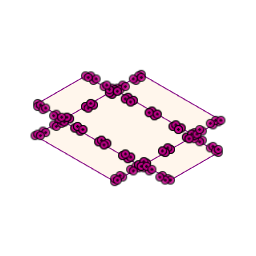
3dBox v7 (Autodesk Fusion 360 design; units mm, degrees)
Autodesk Fusion 360 part; units mm, degrees
sketch "Sketch1" plane through (0, 0, 0) normal (0, 0, 1) x (1, 0, 0) in component "bottom"
  line L0 (0, 100) -> (150, 100)
  line L1 (150, 100) -> (150, 0)
  line L2 (150, 0) -> (0, 0)
  line L3 (0, 0) -> (0, 100)
  line L4 (150, 100) -> (145, 100)
  line L5 (145, 100) -> (145, 90)
  line L6 (145, 90) -> (150, 90)
  line L7 (150, 90) -> (150, 55)
  line L8 (150, 55) -> (145, 55)
  line L9 (145, 55) -> (145, 45)
  line L10 (145, 45) -> (150, 45)
  line L11 (150, 45) -> (150, 10)
  line L12 (150, 10) -> (145, 10)
  line L13 (145, 10) -> (145, 0)
  line L14 (145, 0) -> (150, 0)
  line L15 (75, 100) -> (75, 0) construction
  line L16 (5, 100) -> (5, 90)
  line L17 (5, 90) -> (0, 90)
  line L18 (0, 55) -> (5, 55)
  line L19 (5, 55) -> (5, 45)
  line L20 (5, 45) -> (0, 45)
  line L21 (0, 10) -> (5, 10)
  line L22 (5, 10) -> (5, 0)
  line L23 (5, 0) -> (0, 0)
  line L24 (25, 100) -> (25, 95)
  line L25 (25, 95) -> (35, 95)
  line L26 (35, 95) -> (35, 100)
  line L27 (35, 100) -> (70, 100)
  line L28 (70, 100) -> (70, 95)
  line L29 (70, 95) -> (80, 95)
  line L30 (80, 95) -> (80, 100)
  line L31 (80, 100) -> (115, 100)
  line L32 (115, 100) -> (115, 95)
  line L33 (115, 95) -> (125, 95)
  line L34 (125, 95) -> (125, 100)
  line L35 (125, 100) -> (145, 100)
  line L36 (25, 100) -> (5, 100)
  line L37 (75, 50) -> (103.6625, 50) construction
  line L38 (25, 0) -> (25, 5)
  line L39 (25, 5) -> (35, 5)
  line L40 (35, 5) -> (35, 0)
  line L41 (70, 0) -> (70, 5)
  line L42 (70, 5) -> (80, 5)
  line L43 (80, 5) -> (80, 0)
  line L44 (115, 0) -> (115, 5)
  line L45 (115, 5) -> (125, 5)
  line L46 (125, 5) -> (125, 0)
  dimension "d1" = 150
  dimension "d2" = 100
  dimension "d5" = 5
  dimension "d6" = 5
  dimension "d7" = 5
  dimension "d8" = 5
  dimension "d9" = 5
  dimension "d10" = 5
  dimension "d11" = 100
  dimension "d12" = 10
  dimension "d13" = 10
  dimension "d14" = 10
  dimension "d15" = 5
  dimension "d16" = 5
  dimension "d17" = 5
  dimension "d18" = 5
  dimension "d19" = 5
  dimension "d20" = 5
  dimension "d21" = 10
  dimension "d22" = 10
  dimension "d23" = 10
  dimension "d24" = 140
  dimension "d25" = 20
  dimension "d26" = 20
  constraint horizontal L0
  constraint vertical L1
  constraint horizontal L2
  constraint vertical L3
  constraint coincident L2.end L3.start
  constraint horizontal L4
  constraint perpendicular L4 L5
  constraint perpendicular L5 L6
  constraint perpendicular L6 L7
  constraint perpendicular L7 L8
  constraint perpendicular L8 L9
  constraint perpendicular L7 L10
  constraint perpendicular L8 L11
  constraint perpendicular L11 L12
  constraint perpendicular L12 L13
  constraint perpendicular L13 L14
  constraint equal L7 L11
  constraint coincident L1.end L2.start
  constraint midpoint L0 L15.start
  constraint midpoint L2 L15.end
  constraint symmetric L4.end L15 L16.start
  constraint symmetric L5.end L15 L16.end
  constraint symmetric L6.end L15 L17.end
  constraint symmetric L7.end L15 L18.start
  constraint symmetric L8.end L15 L18.end
  constraint symmetric L9.end L15 L19.end
  constraint symmetric L10.end L15 L20.end
  constraint symmetric L11.end L15 L21.start
  constraint symmetric L12.end L15 L21.end
  constraint symmetric L13.end L15 L22.end
  constraint symmetric L1.end L15 L2.end
  constraint perpendicular L0 L24
  constraint perpendicular L24 L25
  constraint perpendicular L25 L26
  constraint perpendicular L26 L27
  constraint perpendicular L27 L28
  constraint perpendicular L28 L29
  constraint perpendicular L29 L30
  constraint perpendicular L30 L31
  constraint perpendicular L31 L32
  constraint perpendicular L30 L33
  constraint perpendicular L33 L34
  constraint perpendicular L34 L35
  constraint perpendicular L24 L36
  constraint equal L27 L31
  constraint coincident L16.start L36.end
  constraint midpoint L15 L37.start
  constraint perpendicular L1 L37
  constraint symmetric L24.start L37 L38.start
  constraint symmetric L24.end L37 L38.end
  constraint symmetric L25.end L37 L39.end
  constraint symmetric L26.end L37 L40.end
  constraint symmetric L27.end L37 L41.start
  constraint symmetric L28.end L37 L41.end
  constraint symmetric L29.end L37 L42.end
  constraint symmetric L30.end L37 L43.end
  constraint symmetric L31.end L37 L44.start
  constraint symmetric L32.end L37 L44.end
  constraint symmetric L33.end L37 L45.end
  constraint symmetric L34.end L37 L46.end
  measures "d1" distance of L0.start L0.end
  measures "d2" distance of L0.start L2.end
  measures "d5" distance of L0.end L4.end
  measures "d6" distance of L5.end L6.end
  measures "d7" distance of L7.end L8.end
  measures "d8" distance of L9.end L10.end
  measures "d9" distance of L11.end L12.end
  measures "d10" distance of L13.end L1.end
  measures "d11" distance of L0.end L1.end
  measures "d12" distance of L12.end L13.end
  measures "d13" distance of L8.end L9.end
  measures "d14" distance of L4.end L5.end
  measures "d15" distance of L33.end L34.end
  measures "d16" distance of L31.end L32.end
  measures "d17" distance of L29.end L30.end
  measures "d18" distance of L27.end L28.end
  measures "d19" distance of L25.end L26.end
  measures "d20" distance of L24.start L24.end
  measures "d21" distance of L24.end L25.end
  measures "d22" distance of L28.end L29.end
  measures "d23" distance of L32.end L33.end
  measures "d24" distance of L4.end L16.start
  measures "d25" distance of L34.end L4.end
  measures "d26" distance of L24.start L16.start
extrude "Extrude1" add sketch "Sketch1" along normal blind 5 contours L0 L1 L2 L3 L5 L6 L7 L8 L9 L10 L11 L12 L13 L16 L17 L18 L19 L20 L21 L22 L24 L25 L26 L27 L28 L29 L30 L31 L32 L33 L34 L35 L36 L38 L39 L40 L41 L42 L43 L44 L45 L46 makes body 1 in component "bottom"
sketch "Sketch1 (2)" plane through (0, 0, 0) normal (0, 0, 1) x (1, 0, 0) in component "sSide"
  line L0 (115, 0) -> (115, 5)
  line L1 (115, 5) -> (125, 5)
  line L2 (125, 5) -> (125, 0)
  line L3 (125, 0) -> (145, 0)
  line L4 (145, 0) -> (145, 10)
  line L5 (145, 10) -> (150, 10)
  line L6 (150, 10) -> (150, 45)
  line L7 (150, 45) -> (145, 45)
  line L8 (145, 45) -> (145, 55)
  line L9 (145, 55) -> (150, 55)
  line L10 (150, 55) -> (150, 90)
  line L11 (150, 90) -> (145, 90)
  line L12 (145, 90) -> (145, 100)
  line L13 (145, 100) -> (125, 100)
  line L14 (125, 100) -> (125, 95)
  line L15 (125, 95) -> (115, 95)
  line L16 (115, 95) -> (115, 100)
  line L17 (115, 100) -> (80, 100)
  line L18 (80, 100) -> (80, 95)
  line L19 (80, 95) -> (70, 95)
  line L20 (70, 95) -> (70, 100)
  line L21 (70, 100) -> (35, 100)
  line L22 (35, 100) -> (35, 95)
  line L23 (35, 95) -> (25, 95)
  line L24 (25, 95) -> (25, 100)
  line L25 (25, 100) -> (5, 100)
  line L26 (5, 100) -> (5, 90)
  line L27 (5, 90) -> (0, 90)
  line L28 (0, 90) -> (0, 55)
  line L29 (0, 55) -> (5, 55)
  line L30 (5, 55) -> (5, 45)
  line L31 (5, 45) -> (0, 45)
  line L32 (0, 45) -> (0, 10)
  line L33 (0, 10) -> (5, 10)
  line L34 (5, 10) -> (5, 0)
  line L35 (5, 0) -> (25, 0)
  line L36 (25, 0) -> (25, 5)
  line L37 (25, 5) -> (35, 5)
  line L38 (35, 5) -> (35, 0)
  line L39 (35, 0) -> (70, 0)
  line L40 (70, 0) -> (70, 5)
  line L41 (70, 5) -> (80, 5)
  line L42 (80, 5) -> (80, 0)
  line L43 (80, 0) -> (115, 0)
  line L44 (145, 100) -> (200, 100)
  line L45 (200, 100) -> (200, 0)
  line L46 (200, 0) -> (145, 0)
  line L47 (145, 100) -> (150, 100)
  line L48 (150, 100) -> (150, 95)
  line L49 (150, 95) -> (155, 95)
  line L50 (155, 95) -> (155, 100)
  line L51 (155, 100) -> (165, 100)
  line L52 (165, 100) -> (165, 95)
  line L53 (165, 95) -> (185, 95)
  line L54 (185, 95) -> (185, 100)
  line L55 (185, 100) -> (195, 100)
  line L56 (195, 100) -> (195, 95)
  line L57 (195, 95) -> (200, 95)
  line L58 (200, 50) -> (169.7246, 50) construction
  line L59 (195, 5) -> (200, 5)
  line L60 (195, 0) -> (195, 5)
  line L61 (185, 5) -> (185, 0)
  line L62 (165, 5) -> (185, 5)
  line L63 (165, 0) -> (165, 5)
  line L64 (155, 5) -> (155, 0)
  line L65 (150, 5) -> (155, 5)
  line L66 (150, 0) -> (150, 5)
  dimension "d55" = 5
  dimension "d56" = 5
  dimension "d57" = 5
  dimension "d58" = 5
  dimension "d59" = 5
  dimension "d60" = 5
  dimension "d61" = 5
  dimension "d62" = 5
  dimension "d63" = 10
  dimension "d64" = 10
  dimension "d65" = 55
  dimension "d66" = 55
  constraint coincident L12.end L13.start
  constraint perpendicular L12 L44
  constraint perpendicular L3 L45
  constraint coincident L3.end L4.start
  constraint perpendicular L4 L46
  constraint horizontal L47
  constraint perpendicular L47 L48
  constraint perpendicular L48 L49
  constraint perpendicular L47 L50
  constraint perpendicular L50 L51
  constraint perpendicular L47 L52
  constraint perpendicular L52 L53
  constraint perpendicular L53 L54
  constraint perpendicular L54 L55
  constraint perpendicular L55 L56
  constraint perpendicular L56 L57
  constraint midpoint L45 L58.start
  constraint perpendicular L45 L58
  constraint symmetric L47.end L58 L66.start
  constraint symmetric L48.end L58 L65.start
  constraint symmetric L49.end L58 L64.start
  constraint symmetric L50.end L58 L64.end
  constraint symmetric L51.end L58 L63.start
  constraint symmetric L52.end L58 L62.start
  constraint symmetric L53.end L58 L61.start
  constraint symmetric L54.end L58 L61.end
  constraint symmetric L55.end L58 L60.start
  constraint symmetric L56.end L58 L59.start
  constraint symmetric L57.end L58 L59.end
  measures "d55" distance of L12.end L47.end
  measures "d56" distance of L47.end L48.end
  measures "d57" distance of L48.end L49.end
  measures "d58" distance of L49.end L50.end
  measures "d59" distance of L51.end L52.end
  measures "d60" distance of L53.end L54.end
  measures "d61" distance of L55.end L56.end
  measures "d62" distance of L56.end L57.end
  measures "d63" distance of L50.end L51.end
  measures "d64" distance of L54.end L55.end
  measures "d65" distance of L12.end L44.end
  measures "d66" horizontal distance of L12.end L57.end
extrude "Extrude1'" add sketch "Sketch1 (2)" along normal blind 5 separate body contours L4 L5 L6 L7 L8 L9 L10 L11 L12 L44 L45 L46 L47 L48 L49 L50 L51 L52 L53 L54 L55 L56 L57 L59 L60 L61 L62 L63 L64 L65 L66 makes body 2 in component "sSide"
sketch "Sketch1 (3)" plane through (0, 0, 0) normal (0, 0, 1) x (1, 0, 0) in component "lSide"
  line L0 (115, 0) -> (115, 5)
  line L1 (115, 5) -> (125, 5)
  line L2 (125, 5) -> (125, 0)
  line L3 (125, 0) -> (145, 0)
  line L4 (145, 0) -> (145, 10)
  line L5 (145, 10) -> (150, 10)
  line L6 (150, 10) -> (150, 45)
  line L7 (150, 45) -> (145, 45)
  line L8 (145, 45) -> (145, 55)
  line L9 (145, 55) -> (150, 55)
  line L10 (150, 55) -> (150, 90)
  line L11 (150, 90) -> (145, 90)
  line L12 (145, 90) -> (145, 100)
  line L13 (145, 100) -> (125, 100)
  line L14 (125, 100) -> (125, 95)
  line L15 (125, 95) -> (115, 95)
  line L16 (115, 95) -> (115, 100)
  line L17 (115, 100) -> (80, 100)
  line L18 (80, 100) -> (80, 95)
  line L19 (80, 95) -> (70, 95)
  line L20 (70, 95) -> (70, 100)
  line L21 (70, 100) -> (35, 100)
  line L22 (35, 100) -> (35, 95)
  line L23 (35, 95) -> (25, 95)
  line L24 (25, 95) -> (25, 100)
  line L25 (25, 100) -> (5, 100)
  line L26 (5, 100) -> (5, 90)
  line L27 (5, 90) -> (0, 90)
  line L28 (0, 90) -> (0, 55)
  line L29 (0, 55) -> (5, 55)
  line L30 (5, 55) -> (5, 45)
  line L31 (5, 45) -> (0, 45)
  line L32 (0, 45) -> (0, 10)
  line L33 (0, 10) -> (5, 10)
  line L34 (5, 10) -> (5, 0)
  line L35 (5, 0) -> (25, 0)
  line L36 (25, 0) -> (25, 5)
  line L37 (25, 5) -> (35, 5)
  line L38 (35, 5) -> (35, 0)
  line L39 (35, 0) -> (70, 0)
  line L40 (70, 0) -> (70, 5)
  line L41 (70, 5) -> (80, 5)
  line L42 (80, 5) -> (80, 0)
  line L43 (80, 0) -> (115, 0)
  line L44 (145, 100) -> (150, 100)
  line L45 (150, 100) -> (150, 150)
  line L46 (150, 150) -> (0, 150)
  line L47 (0, 150) -> (0, 100)
  line L48 (5, 100) -> (0, 100)
  line L49 (150, 150) -> (150, 145)
  line L50 (150, 145) -> (145, 145)
  line L51 (145, 145) -> (145, 135)
  line L52 (145, 135) -> (150, 135)
  line L53 (150, 135) -> (150, 115)
  line L54 (150, 115) -> (145, 115)
  line L55 (145, 115) -> (145, 105)
  line L56 (145, 105) -> (150, 105)
  line L57 (150, 105) -> (150, 100)
  line L58 (75, 150) -> (75, 127.5364) construction
  line L59 (0, 145) -> (5, 145)
  line L60 (5, 145) -> (5, 135)
  line L61 (5, 135) -> (0, 135)
  line L62 (0, 115) -> (5, 115)
  line L63 (5, 115) -> (5, 105)
  line L64 (5, 105) -> (0, 105)
  dimension "d33" = 50
  dimension "d34" = 150
  dimension "d35" = 10
  dimension "d36" = 10
  dimension "d37" = 5
  dimension "d38" = 5
  dimension "d39" = 5
  dimension "d40" = 5
  dimension "d41" = 50
  dimension "d42" = 5
  constraint coincident L12.end L13.start
  constraint perpendicular L12 L44
  constraint perpendicular L11 L45
  constraint perpendicular L28 L46
  constraint perpendicular L27 L47
  constraint coincident L25.end L26.start
  constraint perpendicular L47 L48
  constraint perpendicular L46 L49
  constraint perpendicular L49 L50
  constraint perpendicular L50 L51
  constraint perpendicular L51 L52
  constraint perpendicular L52 L53
  constraint perpendicular L53 L54
  constraint perpendicular L52 L55
  constraint perpendicular L53 L56
  constraint perpendicular L52 L57
  constraint equal L44 L48
  constraint equal L49 L57
  constraint coincident L45.end L46.start
  constraint midpoint L46 L58.start
  constraint perpendicular L46 L58
  constraint symmetric L49.end L58 L59.start
  constraint symmetric L50.end L58 L59.end
  constraint symmetric L51.end L58 L60.end
  constraint symmetric L52.end L58 L61.end
  constraint symmetric L53.end L58 L62.start
  constraint symmetric L54.end L58 L62.end
  constraint symmetric L55.end L58 L63.end
  constraint symmetric L56.end L58 L64.end
  measures "d33" distance of L20.end L46
  measures "d34" distance of L45.end L46.end
  measures "d35" distance of L50.end L51.end
  measures "d36" distance of L54.end L55.end
  measures "d37" distance of L49.end L50.end
  measures "d38" distance of L51.end L52.end
  measures "d39" distance of L53.end L54.end
  measures "d40" distance of L55.end L56.end
  measures "d41" distance of L45.end L44.end
  measures "d42" distance of L56.end L44.end
extrude "Extrude1''" add sketch "Sketch1 (3)" along normal blind 5 separate body contours L13 L14 L15 L16 L17 L18 L19 L20 L21 L22 L23 L24 L25 L44 L45 L46 L47 L48 L49 L50 L51 L52 L53 L54 L55 L56 L57 L59 L60 L61 L62 L63 L64 makes body 3 in component "lSide"
copy_body "CopyPasteBodies1" bodies 3 makes body 4 in component "lSide"
move_body "Move1" bodies 4 to x (1, 0, 0) y (0, 1, 0) z (0, 0, 1) at (-1.8416, -152.2425, 0) in component "lSide"
move_body "Move2" bodies 4 to x (-1, 0, 0) y (0, -1, 0) z (0, 0, 1) at (0, 0, 0) in component "lSide"
move_body "Move3" bodies 4 to x (1, 0, 0) y (0, 1, 0) z (0, 0, 1) at (148.1584, -52.2425, 0) in component "lSide"
copy_body "CopyPasteBodies1'" bodies 2 makes body 5 in component "sSide"
move_body "Move1'" bodies 5 to x (-1, 0, 0) y (0, -1, 0) z (0, 0, 1) at (0, 0, 0) in component "sSide"
move_body "Move2'" bodies 5 to x (1, 0, 0) y (0, 1, 0) z (0, 0, 1) at (150, 100, 0) in component "sSide"
sketch "Sketch1 (4)" plane through (0, 0, 0) normal (0, 0, 1) x (1, 0, 0) in component "exportDXF"
  line L0 (0, -50) -> (150, -50)
  line L1 (150, -50) -> (150, -45)
  line L2 (150, -45) -> (145, -45)
  line L3 (145, -45) -> (145, -35)
  line L4 (145, -35) -> (150, -35)
  line L5 (150, -35) -> (150, -15)
  line L6 (150, -15) -> (145, -15)
  line L7 (145, -15) -> (145, -5)
  line L8 (145, -5) -> (150, -5)
  line L9 (150, -5) -> (150, 0)
  line L10 (150, 0) -> (125, 0)
  line L11 (125, 0) -> (125, 5)
  line L12 (125, 5) -> (115, 5)
  line L13 (115, 5) -> (115, 0)
  line L14 (115, 0) -> (80, 0)
  line L15 (80, 0) -> (80, 5)
  line L16 (80, 5) -> (70, 5)
  line L17 (70, 5) -> (70, 0)
  line L18 (70, 0) -> (35, 0)
  line L19 (35, 0) -> (35, 5)
  line L20 (35, 5) -> (25, 5)
  line L21 (25, 5) -> (25, 0)
  line L22 (25, 0) -> (0, 0)
  line L23 (0, 0) -> (0, -5)
  line L24 (0, -5) -> (5, -5)
  line L25 (5, -5) -> (5, -15)
  line L26 (5, -15) -> (0, -15)
  line L27 (0, -15) -> (0, -35)
  line L28 (0, -35) -> (5, -35)
  line L29 (5, -35) -> (5, -45)
  line L30 (5, -45) -> (0, -45)
  line L31 (0, -45) -> (0, -50)
  line L32 (115, 0) -> (115, 5)
  line L33 (115, 5) -> (125, 5)
  line L34 (125, 5) -> (125, 0)
  line L35 (125, 0) -> (145, 0)
  line L36 (145, 0) -> (145, 10)
  line L37 (145, 10) -> (150, 10)
  line L38 (150, 10) -> (150, 45)
  line L39 (150, 45) -> (145, 45)
  line L40 (145, 45) -> (145, 55)
  line L41 (145, 55) -> (150, 55)
  line L42 (150, 55) -> (150, 90)
  line L43 (150, 90) -> (145, 90)
  line L44 (145, 90) -> (145, 100)
  line L45 (145, 100) -> (125, 100)
  line L46 (125, 100) -> (125, 95)
  line L47 (125, 95) -> (115, 95)
  line L48 (115, 95) -> (115, 100)
  line L49 (115, 100) -> (80, 100)
  line L50 (80, 100) -> (80, 95)
  line L51 (80, 95) -> (70, 95)
  line L52 (70, 95) -> (70, 100)
  line L53 (70, 100) -> (35, 100)
  line L54 (35, 100) -> (35, 95)
  line L55 (35, 95) -> (25, 95)
  line L56 (25, 95) -> (25, 100)
  line L57 (25, 100) -> (5, 100)
  line L58 (5, 100) -> (5, 90)
  line L59 (5, 90) -> (0, 90)
  line L60 (0, 90) -> (0, 55)
  line L61 (0, 55) -> (5, 55)
  line L62 (5, 55) -> (5, 45)
  line L63 (5, 45) -> (0, 45)
  line L64 (0, 45) -> (0, 10)
  line L65 (0, 10) -> (5, 10)
  line L66 (5, 10) -> (5, 0)
  line L67 (5, 0) -> (25, 0)
  line L68 (25, 0) -> (25, 5)
  line L69 (25, 5) -> (35, 5)
  line L70 (35, 5) -> (35, 0)
  line L71 (35, 0) -> (70, 0)
  line L72 (70, 0) -> (70, 5)
  line L73 (70, 5) -> (80, 5)
  line L74 (80, 5) -> (80, 0)
  line L75 (80, 0) -> (115, 0)
  line L76 (145, 0) -> (150, 0)
  line L77 (150, 0) -> (150, 5)
  line L78 (150, 5) -> (155, 5)
  line L79 (155, 5) -> (155, 0)
  line L80 (155, 0) -> (165, 0)
  line L81 (165, 0) -> (165, 5)
  line L82 (165, 5) -> (185, 5)
  line L83 (185, 5) -> (185, 0)
  line L84 (185, 0) -> (195, 0)
  line L85 (195, 0) -> (195, 5)
  line L86 (195, 5) -> (200, 5)
  line L87 (200, 5) -> (200, 95)
  line L88 (200, 95) -> (195, 95)
  line L89 (195, 95) -> (195, 100)
  line L90 (195, 100) -> (185, 100)
  line L91 (185, 100) -> (185, 95)
  line L92 (185, 95) -> (165, 95)
  line L93 (165, 95) -> (165, 100)
  line L94 (165, 100) -> (155, 100)
  line L95 (155, 100) -> (155, 95)
  line L96 (155, 95) -> (150, 95)
  line L97 (150, 95) -> (150, 100)
  line L98 (150, 100) -> (145, 100)
  line L99 (145, 100) -> (145, 90)
  line L100 (145, 90) -> (150, 90)
  line L101 (150, 90) -> (150, 55)
  line L102 (150, 55) -> (145, 55)
  line L103 (145, 55) -> (145, 45)
  line L104 (145, 45) -> (150, 45)
  line L105 (150, 45) -> (150, 10)
  line L106 (150, 10) -> (145, 10)
  line L107 (145, 10) -> (145, 0)
  line L108 (150, 150) -> (0, 150)
  line L109 (0, 150) -> (0, 145)
  line L110 (0, 145) -> (5, 145)
  line L111 (5, 145) -> (5, 135)
  line L112 (5, 135) -> (0, 135)
  line L113 (0, 135) -> (0, 115)
  line L114 (0, 115) -> (5, 115)
  line L115 (5, 115) -> (5, 105)
  line L116 (5, 105) -> (0, 105)
  line L117 (0, 105) -> (0, 100)
  line L118 (0, 100) -> (25, 100)
  line L119 (25, 100) -> (25, 95)
  line L120 (25, 95) -> (35, 95)
  line L121 (35, 95) -> (35, 100)
  line L122 (35, 100) -> (70, 100)
  line L123 (70, 100) -> (70, 95)
  line L124 (70, 95) -> (80, 95)
  line L125 (80, 95) -> (80, 100)
  line L126 (80, 100) -> (115, 100)
  line L127 (115, 100) -> (115, 95)
  line L128 (115, 95) -> (125, 95)
  line L129 (125, 95) -> (125, 100)
  line L130 (125, 100) -> (150, 100)
  line L131 (150, 100) -> (150, 105)
  line L132 (150, 105) -> (145, 105)
  line L133 (145, 105) -> (145, 115)
  line L134 (145, 115) -> (150, 115)
  line L135 (150, 115) -> (150, 135)
  line L136 (150, 135) -> (145, 135)
  line L137 (145, 135) -> (145, 145)
  line L138 (145, 145) -> (150, 145)
  line L139 (150, 145) -> (150, 150)
  line L140 (5, 100) -> (0, 100)
  line L141 (0, 100) -> (0, 95)
  line L142 (0, 95) -> (-5, 95)
  line L143 (-5, 95) -> (-5, 100)
  line L144 (-5, 100) -> (-15, 100)
  line L145 (-15, 100) -> (-15, 95)
  line L146 (-15, 95) -> (-35, 95)
  line L147 (-35, 95) -> (-35, 100)
  line L148 (-35, 100) -> (-45, 100)
  line L149 (-45, 100) -> (-45, 95)
  line L150 (-45, 95) -> (-50, 95)
  line L151 (-50, 95) -> (-50, 5)
  line L152 (-50, 5) -> (-45, 5)
  line L153 (-45, 5) -> (-45, 0)
  line L154 (-45, 0) -> (-35, 0)
  line L155 (-35, 0) -> (-35, 5)
  line L156 (-35, 5) -> (-15, 5)
  line L157 (-15, 5) -> (-15, 0)
  line L158 (-15, 0) -> (-5, 0)
  line L159 (-5, 0) -> (-5, 5)
  line L160 (-5, 5) -> (0, 5)
  line L161 (0, 5) -> (0, 0)
  line L162 (0, 0) -> (5, 0)
  line L163 (5, 0) -> (5, 10)
  line L164 (5, 10) -> (0, 10)
  line L165 (0, 10) -> (0, 45)
  line L166 (0, 45) -> (5, 45)
  line L167 (5, 45) -> (5, 55)
  line L168 (5, 55) -> (0, 55)
  line L169 (0, 55) -> (0, 90)
  line L170 (0, 90) -> (5, 90)
  line L171 (5, 90) -> (5, 100)
component "bottom" placed x (1, 0, 0) y (0, 1, 0) z (0, 0, 1) at (0, 0, 0)
component "sSide" placed x (1, 0, 0) y (0, 1, 0) z (0, 0, 1) at (0, 0, 0)
component "lSide" placed x (1, 0, 0) y (0, 1, 0) z (0, 0, 1) at (0, 0, 0)
component "exportDXF" placed x (1, 0, 0) y (0, 1, 0) z (0, 0, 1) at (0, 0, 0)
equation "d6 = d5"
equation "d7 = d5"
equation "d8 = d5"
equation "d9 = d5"
equation "d10 = d5"
equation "d11 = d2"
equation "d12 = d14"
equation "d13 = d14"
equation "d15 = d5"
equation "d16 = d5"
equation "d17 = d5"
equation "d18 = d5"
equation "d19 = d5"
equation "d20 = d5"
equation "d21 = d14"
equation "d22 = d14"
equation "d23 = d14"
equation "d26 = d25"
